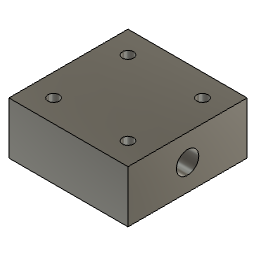
linear_rail_(actuator) v15 (Autodesk Fusion 360 archive; units mm, degrees)
design "Carrige"
Autodesk Fusion 360 part; units mm, degrees
sketch "Sketch1" plane through (0, 0, 0) normal (0, 0, 1) x (1, 0, 0)
  circle A0 centre (26, 26) radius 1.5
  circle A1 centre (6, 6) radius 1.5
  circle A2 centre (6, 26) radius 1.5
  line L0 (0, 0) -> (32, 0)
  circle A3 centre (26, 6) radius 1.5
  line L1 (32, 32) -> (0, 32)
  line L2 (0, 32) -> (0, 0)
  line L3 (32, 0) -> (32, 32)
  dimension "d5" = 20
  dimension "d6" = -20
  dimension "d7" = 32
  dimension "d8" = 32
  dimension "d9" = 3
  dimension "d10" = 6
  dimension "d11" = 6
  constraint horizontal L0
  constraint vertical L3
  constraint horizontal L1
  constraint vertical L2
  constraint coincident L0.start L2.end
  measures "d7" distance of L0.start L0.end
  measures "d8" distance of L1.end L0.start
  measures "d9" diameter of A2
  measures "d10" distance of A2.centre L1
  measures "d11" distance of A2.centre L2
extrude "Extrude1" add sketch "Sketch1" along normal blind 14
sketch "Sketch2" plane through (32, 0, 0) normal (1, 0, 0) x (0, 1, 0)
  line L0 (0, 0) -> (32, 0)
  line L1 (32, 0) -> (32, 14)
  line L2 (32, 14) -> (0, 14)
  line L3 (0, 14) -> (0, 0)
  line L4 (16, 14) -> (16, 0) construction
  line L5 (0, 7) -> (32, 7) construction
  circle A0 centre (16, 7) radius 3
  dimension "d14" = 6
  constraint midpoint L2 L4.start
  constraint midpoint L0 L4.end
  constraint midpoint L3 L5.start
  constraint midpoint L1 L5.end
  constraint midpoint L4 A0.centre
  measures "d14" diameter of A0
extrude "Extrude2" cut sketch "Sketch2" against normal up to surface (32 mm away) contours A0
